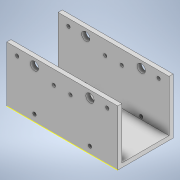
# Autodesk Inventor part: シリンダーボックス
Saved by Autodesk Inventor 2022 (Build 260153070, 153G)
## iProperties
Created: 2022-10-17
Part Number: シリンダーボックス
Material: 一般
Document SubType Name: Modeling
Designer: hirok
Density: 1 g/cm^3
Appearance: 既定
Author: hirok
Autodesk Inventor part; units mm, degrees
ref_plane "YZ Plane" through (0, 0, 0) normal (1, 0, 0) x (0, 1, 0)
ref_plane "XZ Plane" through (0, 0, 0) normal (0, 1, 0) x (-1, 0, 0)
ref_plane "XY Plane" through (0, 0, 0) normal (0, 0, 1) x (1, 0, 0)
sketch "スケッチ1" plane through (0, 0, 0) normal (0, 0, 1) x (1, 0, 0)
  line L0 (0, 0) -> (80, 0)
  line L1 (80, 0) -> (80, 40)
  line L2 (80, 40) -> (0, 40)
  line L3 (0, 40) -> (0, 0)
  dimension "d0" = 80
  dimension "d1" = 40
  constraints: 8 end point, 2 parallel, 1 horizontal, 1 perpendicular
  measures "d0" distance of L0.start L0.end
  measures "d1" distance of L0.end L1.end
extrude "押し出し1" add sketch "スケッチ1" along normal blind 40
sketch "スケッチ2" plane through (80, 0, 0) normal (1, 0, 0) x (0, 0, -1)
  line L0 (0, 40) -> (-40, 40) projected
  line L1 (-37, 40) -> (-3, 40)
  line L2 (-3, 40) -> (-3, 3)
  line L3 (-3, 3) -> (-37, 3)
  line L4 (-37, 3) -> (-37, 40)
  line L5 (-40, 0) -> (-40, 40) projected
  line L6 (0, 0) -> (0, 40) projected
  line L7 (0, 0) -> (-40, 0) projected
  dimension "d4" = 3
  dimension "d5" = 3
  dimension "d6" = 3
  constraints: 8 end point, 2 parallel, 1 horizontal, 1 perpendicular, 1 point on line
  measures "d4" distance between parallel lines of L4 L5
  measures "d5" distance between parallel lines of L6 L2
  measures "d6" distance between parallel lines of L7 L3
extrude "押し出し2" cut sketch "スケッチ2" against normal through all contours L2 L3 L4 L0
sketch "スケッチ3" plane through (0, 0, 40) normal (0, 0, 1) x (1, 0, 0)
  line L0 (0, 40) -> (80, 40) projected
  line L1 (40, 40) -> (40, 0)
  point P0 (0, 0)
  point P1 (20, 35)
  point P2 (60, 35)
  dimension "d9" = 5
  dimension "d10" = 20
  constraints: 2 end point, 1 midpoint, 1 symmetric about line, 1 vertical
  measures "d9" distance from line of point (20, 35) L0
  measures "d10" distance from line of L1 point (20, 35)
hole "穴1" at (20, 35, 40) at (60, 35, 40) direction (0, 0, -1) diameter 6 end through all
sketch "スケッチ4" plane through (0, 0, 40) normal (0, 0, 1) x (1, 0, 0)
  line L0 (0, 40) -> (80, 40) projected
  line L1 (40, 40) -> (40, 0)
  point P0 (0, 0)
  point P1 (34, 30)
  point P2 (46, 30)
  dimension "d18" = 6
  dimension "d19" = 10
  constraints: 2 end point, 1 midpoint, 1 symmetric about line, 1 vertical
  measures "d18" distance from line of L1 point (34, 30)
  measures "d19" distance from line of point (34, 30) L0
hole "穴2" at (34, 30, 40) at (46, 30, 40) direction (0, 0, -1) diameter 2.4 end through all clearance for "Countersunk Flat Head Screw ISO 2009/7046" size "M2" standard "ISO"
sketch "スケッチ5" plane through (0, 0, 0) normal (0, -1, 0) x (1, 0, 0)
  line L0 (80, 40) -> (0, 40) projected
  line L1 (40, 40) -> (40, 10)
  point P0 (0, 0)
  constraints: 2 end point, 1 midpoint, 1 vertical
sketch "スケッチ6" plane through (0, 0, 40) normal (0, 0, 1) x (1, 0, 0)
  line L0 (80, 40) -> (0, 40) projected
  line L1 (40, 40) -> (40, 0)
  line L2 (0, 0) -> (80, 0) projected
  circle A0 centre (20, 35) radius 3 projected
  point P0 (20, 5)
  point P1 (60, 5)
  dimension "d27" = 20
  dimension "d28" = 30
  constraints: 2 end point, 2 midpoint, 1 symmetric about line
  measures "d27" distance from line of L1 point (20, 5)
  measures "d28" distance of point (20, 5) A0.centre
hole "穴3" at (20, 5, 40) at (60, 5, 40) direction (0, 0, -1) diameter 2.459 depth 3 thread size "M3x0.5" class "6H" standard "ISO Metric profile"
sketch "スケッチ7" plane through (0, 0, 0) normal (0, 0, -1) x (-1, 0, 0)
  line L0 (-80, 40) -> (0, 40) projected
  line L1 (-40, 40) -> (-40, 0)
  line L2 (0, 0) -> (-80, 0) projected
  circle A0 centre (-60, 35) radius 3 projected
  point P0 (-60, 5)
  point P1 (-20, 5)
  dimension "d36" = 20
  dimension "d37" = 30
  constraints: 2 end point, 2 midpoint, 1 symmetric about line
  measures "d36" distance from line of L1 point (-60, 5)
  measures "d37" distance of point (-60, 5) A0.centre
hole "穴4" at (60, 5, 0) at (20, 5, 0) direction (0, 0, 1) diameter 2.459 depth 3 thread size "M3x0.5" class "6H" standard "ISO Metric profile"
sketch "スケッチ8" plane through (0, 0, 0) normal (0, 0, -1) x (-1, 0, 0)
  line L0 (-80, 40) -> (0, 40) projected
  line L1 (-40, 40) -> (-40, 3)
  line L2 (-80, 3) -> (0, 3) projected
  point P0 (0, 0)
  point P1 (-72.5, 35)
  point P2 (-7.5, 35)
  dimension "d45" = 5
  dimension "d46" = 32.5
  constraints: 2 end point, 2 midpoint, 1 symmetric about line
  measures "d45" distance from line of point (-72.5, 35) L0
  measures "d46" distance from line of L1 point (-72.5, 35)
hole "穴5" at (72.5, 35, 0) at (7.5, 35, 0) direction (0, 0, 1) diameter 2.459 depth 3 thread size "M3x0.5" class "6H" standard "ISO Metric profile"
sketch "スケッチ9" plane through (0, 0, 40) normal (0, 0, 1) x (1, 0, 0)
  circle A0 centre (7.5, 35) radius 1.2295 projected
  circle A1 centre (72.5, 35) radius 1.2295 projected
  point P0 (0, 0)
  constraints: 2 coincident
hole "穴6" at (7.5, 35, 40) at (72.5, 35, 40) direction (0, 0, -1) diameter 2.459 depth 3 thread size "M3x0.5" class "6H" standard "ISO Metric profile"
